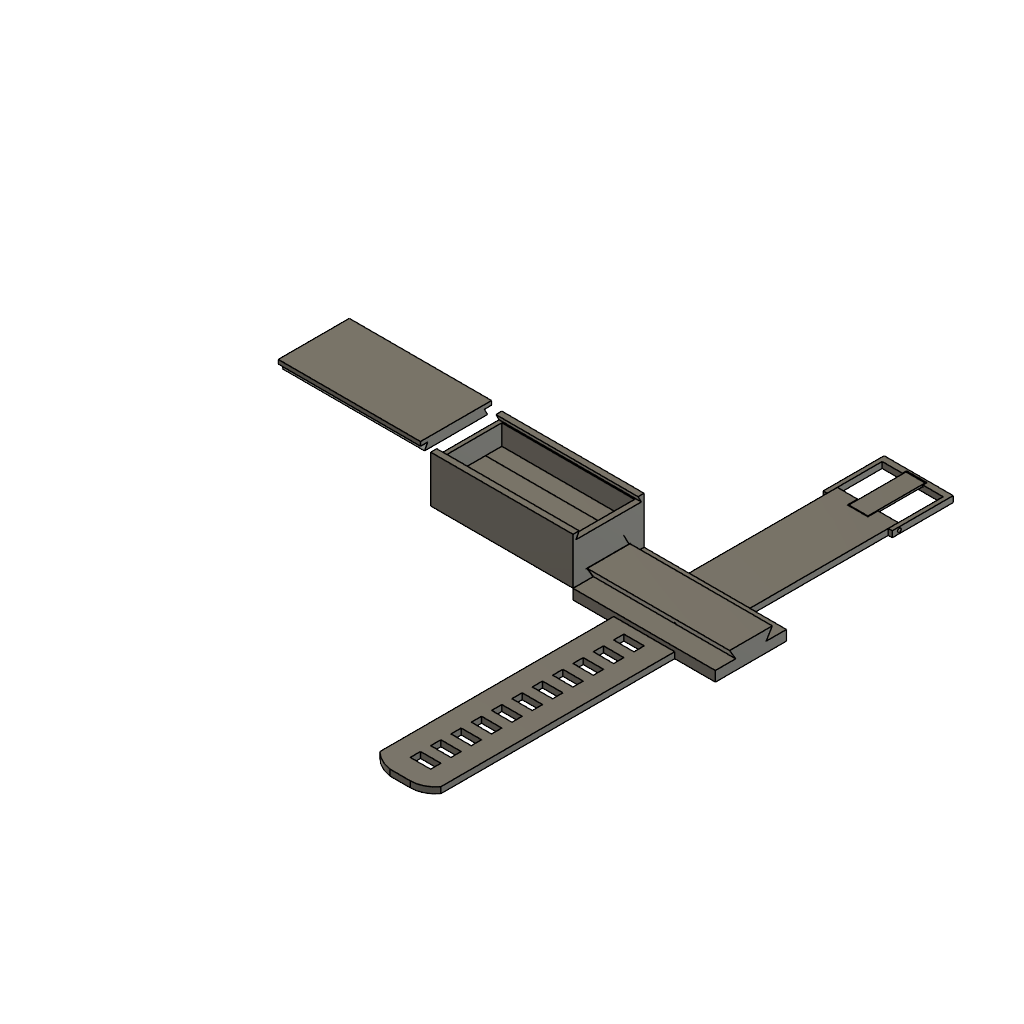
Wristband and components model 2 (Autodesk Fusion 360 design; units mm, degrees)
part number: 2026-09-06-09-34-06-070
Autodesk Fusion 360 part; units mm, degrees
note: some values were not read from the file. Chosen so that the rebuilt part matches the saved one: which bodies a step acts on. Set by a fixed rule: which sketch regions a step uses.
sketch "Sketch1" plane through (0, 0, 0) normal (0, 1, 0) x (1, 0, 0)
  line L0 (0, 35) -> (0, 0)
  line L1 (0, 35) -> (70, 35)
  line L2 (70, 35) -> (70, 0)
  line L3 (70, 0) -> (0, 0)
  constraint vertical L0
  constraint coincident L0.end L3.end
  constraint perpendicular L0 L1
  constraint perpendicular L1 L2
  constraint perpendicular L0 L3
extrude "Extrude1" add sketch "Sketch1" along normal blind 5 makes body 1
sketch "Sketch2" plane through (0, 0, 0) normal (1, 0, 0) x (0, 0, -1)
  line L0 (10, 5) -> (7, 10)
  line L1 (7, 10) -> (28, 10)
  line L2 (28, 10) -> (25, 5)
  line L3 (25, 5) -> (10, 5)
  constraint horizontal L1
  constraint parallel L1 L3
extrude "Extrude2" add sketch "Sketch2" along normal blind 70 bodies 1
sketch "Sketch3" plane through (0, 0, 0) normal (1, 0, 0) x (0, 0, -1)
  line L0 (9.85, 5) -> (6.9, 10)
  line L1 (6.9, 10) -> (6.4, 10.1)
  line L2 (6.4, 10.1) -> (28.25, 10.1)
  line L3 (28.25, 10.1) -> (28.05, 10)
  line L4 (28.05, 10) -> (25.177, 5.0231)
  line L5 (25.177, 5.0231) -> (35, 5.0231)
  line L6 (35, 5.0231) -> (35, 15)
  line L7 (35, 15) -> (0, 15)
  line L8 (0, 15) -> (0, 5.0231)
  line L9 (0, 5.0231) -> (9.85, 5)
  constraint horizontal L2
  constraint parallel L2 L5
  constraint perpendicular L2 L6
  constraint perpendicular L6 L7
  constraint perpendicular L7 L8
extrude "Extrude3" add sketch "Sketch3" against normal blind 70 separate body makes body 2
move_body "Move1" bodies 2 to x (1, 0, 0) y (0, 1, 0) z (0, 0, 1) at (-9, 0, 0)
move_body "Move2" bodies 2 to x (1, 0, 0) y (0, 1, 0) z (0, 0, 1) at (79, 0, 0)
ref_plane "WorkPlane1" through (0, 5, 0) normal (0, 1, 0) x (0, 0, 1)
sketch "Sketch4" plane through (0, 5, 0) normal (0, 1, 0) x (1, 0, 0)
  arc A0 (40, 10) -> (40.5, 9.5) centre (40.6858, 10.1858) ccw
  arc A1 (40.5, 9.5) -> (40.9, 10) centre (40.2285, 10.1272) ccw
  line L0 (40, 10) -> (40.9, 10)
  constraint horizontal L0
extrude "Extrude4" cut sketch "Sketch4" along normal blind 1 bodies 1 2
move_body "Move3" bodies 2 to x (1, 0, 0) y (0, 1, 0) z (0, 0, 1) at (-75, 0, 0)
sketch "Sketch5" plane through (0, 0, 0) normal (1, 0, 0) x (0, 0, -1)
  line L0 (7.5, 10.1) -> (10, 15)
  line L1 (10, 15) -> (25, 15)
  line L2 (25, 15) -> (27.5, 10.1)
  line L3 (27.5, 10.1) -> (7.5, 10.1)
  constraint horizontal L1
  constraint parallel L1 L3
extrude "Extrude5" cut sketch "Sketch5" against normal blind 75 bodies 2 makes body 3 at (-28.3333, 15, -6.6667)
sketch "Sketch7" plane through (0, 0, 0) normal (1, 0, 0) x (0, 0, -1)
  line L0 (0, 25) -> (35, 25)
  line L1 (27.5, 10.1) -> (7.5, 10.1)
  line L2 (7.5, 10.1) -> (10, 15)
  line L3 (10, 15) -> (0, 15)
  line L4 (0, 15) -> (0, 25)
  line L5 (35, 25) -> (35, 14.9709)
  line L6 (35, 14.9709) -> (25, 14.9709)
  line L7 (25, 14.9709) -> (27.5, 10.1)
  constraint perpendicular L0 L4
  constraint perpendicular L0 L5
  constraint perpendicular L5 L6
move_body "Move4" bodies 2 3 to x (1, 0, 0) y (0, 1, 0) z (0, 0, 1) at (5, 0, 0)
extrude "Extrude6" add sketch "Sketch7" against normal blind 70 bodies 1 3
combine "Combine1" operation add target body 3 tool bodies 2
sketch "Sketch8" plane through (0, 25, 0) normal (0, 1, 0) x (-1, 0, 0)
  line L0 (0, 0) -> (0, -35)
  line L1 (0, -35) -> (70, -35)
  line L2 (70, -35) -> (70, 0)
  line L3 (70, 0) -> (0, 0)
  line L4 (68, -33) -> (2.749, -33)
  line L5 (2.749, -33) -> (2.749, -2.8)
  line L6 (2.749, -2.8) -> (68, -2.8)
  line L7 (68, -2.8) -> (68, -33)
  dimension "d16" = 30.2
  constraint horizontal L4
  constraint vertical L5
  constraint horizontal L6
  constraint vertical L7
  measures "d16" distance of L4.start L6.end
extrude "Extrude7" cut sketch "Sketch8" against normal blind 10 contours L4 L5 L6 L7 bodies 3
sketch "Sketch9" plane through (0, 0, 0) normal (1, 0, 0) x (0, 0, -1)
  line L0 (0, 25) -> (0, 28)
  line L1 (0, 28) -> (3, 28)
  line L2 (3, 28) -> (1.5, 25)
  line L3 (1.5, 25) -> (0, 25)
  line L4 (35, 25) -> (35, 28)
  line L5 (35, 28) -> (32, 28)
  line L6 (32, 28) -> (33.6009, 25)
  line L7 (33.6009, 25) -> (35, 25)
  constraint vertical L0
  constraint perpendicular L0 L1
  constraint perpendicular L0 L3
  constraint perpendicular L3 L4
  constraint perpendicular L4 L5
  constraint perpendicular L4 L7
extrude "Extrude8" add sketch "Sketch9" against normal blind 70 bodies 3
sketch "Sketch12" plane through (0, 0, 0) normal (1, 0, 0) x (0, 0, -1)
  line L0 (2, 25) -> (3.5, 28)
  line L1 (3.5, 28) -> (0, 28)
  line L2 (0, 28) -> (0, 30)
  line L3 (0, 30) -> (35, 30)
  line L4 (35, 30) -> (35, 28)
  line L5 (35, 28) -> (31.5, 28)
  line L6 (31.5, 28) -> (33, 25)
  line L7 (33, 25) -> (2, 25)
  constraint horizontal L1
  constraint perpendicular L1 L2
  constraint perpendicular L2 L3
  constraint perpendicular L3 L4
  constraint perpendicular L4 L5
  constraint perpendicular L4 L7
extrude "Extrude9" add sketch "Sketch12" against normal blind 70 separate body makes body 4
move_body "Move5" bodies 4 to x (1, 0, 0) y (0, 1, 0) z (0, 0, 1) at (70, 0, 0)
move_body "Move6" bodies 4 to x (1, 0, 0) y (0, 1, 0) z (0, 0, 1) at (-145, 0, 0)
sketch "Sketch13" plane through (0, 0, 0) normal (0, 1, 0) x (1, 0, 0)
  line L0 (20, 0) -> (50, 0)
  line L1 (50, 0) -> (50, -120)
  line L2 (50, -120) -> (20, -120)
  line L3 (20, -120) -> (20, 0)
  line L4 (20, 35) -> (50, 35)
  line L5 (50, 35) -> (50, 110)
  line L6 (50, 110) -> (20, 110)
  line L7 (20, 110) -> (20, 35)
  constraint horizontal L0
  constraint vertical L1
  constraint horizontal L2
  constraint vertical L3
  constraint horizontal L4
  constraint vertical L5
  constraint horizontal L6
  constraint vertical L7
extrude "Extrude10" add sketch "Sketch13" along normal blind 3 bodies 1
sketch "Sketch14" plane through (0, 3, 0) normal (0, 1, 0) x (-1, 0, 0)
  line L0 (-40.9, -10) -> (-40, -10)
  line L1 (-40, -10) -> (0, -10)
  line L2 (0, -10) -> (0, 0)
  line L3 (0, 0) -> (-70, 0)
  line L4 (-70, 0) -> (-70, -10)
  line L5 (-30, 5) -> (-40, 5)
  line L6 (-40, 5) -> (-40, 10)
  line L7 (-40, 10) -> (-30, 10)
  line L8 (-30, 10) -> (-30, 5)
  line L9 (-30, 15) -> (-40, 15)
  line L10 (-40, 15) -> (-40, 20)
  line L11 (-40, 20) -> (-30, 20)
  line L12 (-30, 20) -> (-30, 15)
  line L13 (-30, 25) -> (-40, 25)
  line L14 (-40, 25) -> (-40, 30)
  line L15 (-40, 30) -> (-30, 30)
  line L16 (-30, 30) -> (-30, 25)
  line L17 (-30, 35) -> (-40, 35)
  line L18 (-40, 35) -> (-40, 40)
  line L19 (-40, 40) -> (-30, 40)
  line L20 (-30, 40) -> (-30, 35)
  line L21 (-30, 45) -> (-40, 45)
  line L22 (-40, 45) -> (-40, 50)
  line L23 (-40, 50) -> (-30, 50)
  line L24 (-30, 50) -> (-30, 45)
  line L25 (-30, 55) -> (-40, 55)
  line L26 (-40, 55) -> (-40, 60)
  line L27 (-40, 60) -> (-30, 60)
  line L28 (-30, 60) -> (-30, 55)
  line L29 (-30, 65) -> (-40, 65)
  line L30 (-40, 65) -> (-40, 70)
  line L31 (-40, 70) -> (-30, 70)
  line L32 (-30, 70) -> (-30, 65)
  line L33 (-30, 75) -> (-40, 75)
  line L34 (-40, 75) -> (-40, 80)
  line L35 (-40, 80) -> (-30, 80)
  line L36 (-30, 80) -> (-30, 75)
  line L37 (-30, 85) -> (-40, 85)
  line L38 (-40, 85) -> (-40, 90)
  line L39 (-40, 90) -> (-30, 90)
  line L40 (-30, 90) -> (-30, 85)
  line L41 (-30, 95) -> (-40, 95)
  line L42 (-40, 95) -> (-40, 100)
  line L43 (-40, 100) -> (-30, 100)
  line L44 (-30, 100) -> (-30, 95)
  line L45 (-30, 105) -> (-40, 105)
  line L46 (-40, 105) -> (-40, 110)
  line L47 (-40, 110) -> (-30, 110)
  line L48 (-30, 110) -> (-30, 105)
  arc A0 (-20, 115) -> (-30, 120) centre (-32.5, 102.5) ccw
  line L49 (-20, 115) -> (-20, 120)
  line L50 (-40, 120) -> (-50, 120)
  arc A1 (-39, 120) -> (-50, 115) centre (-37.9615, 103.1154) ccw
  line L51 (-70, -10) -> (-40.9, -10)
  constraint perpendicular L5 L6
  constraint perpendicular L5 L8
  constraint horizontal L9
  constraint vertical L10
  constraint horizontal L11
  constraint vertical L12
  constraint horizontal L13
  constraint vertical L14
  constraint horizontal L15
  constraint vertical L16
  constraint horizontal L17
  constraint vertical L18
  constraint horizontal L19
  constraint vertical L20
  constraint horizontal L21
  constraint vertical L22
  constraint horizontal L23
  constraint vertical L24
  constraint horizontal L25
  constraint vertical L26
  constraint horizontal L27
  constraint vertical L28
  constraint horizontal L29
  constraint vertical L30
  constraint horizontal L31
  constraint vertical L32
  constraint horizontal L33
  constraint vertical L34
  constraint horizontal L35
  constraint vertical L36
  constraint horizontal L37
  constraint vertical L38
  constraint horizontal L39
  constraint vertical L40
  constraint horizontal L41
  constraint vertical L42
  constraint horizontal L43
  constraint vertical L44
  constraint horizontal L45
  constraint vertical L46
  constraint horizontal L47
  constraint vertical L48
extrude "Extrude11" cut sketch "Sketch14" against normal blind 17 contours L5 L6 L7 L8 | L9 L10 L11 L12 | L13 L14 L15 L16 | L17 L18 L19 L20 | L21 L22 L23 L24 | L25 L26 L27 L28 | L29 L30 L31 L32 | L33 L34 L35 L36 | L37 L38 L39 L40 | L41 L42 L43 L44 | L45 L46 L47 L48 bodies 1
sketch "Sketch15" plane through (0, 0, 0) normal (0, 1, 0) x (1, 0, 0)
  line L0 (20, -120) -> (30, -120)
  arc A0 (20, -115) -> (30, -120) centre (32.5, -102.5) ccw
  line L1 (20, -115) -> (20, -120)
  line L2 (50, -115) -> (50, -120)
  line L3 (50, -120) -> (40, -120)
  arc A1 (40, -120) -> (50, -115) centre (40, -107.5) ccw
  constraint horizontal L0
  constraint perpendicular L0 L1
  constraint perpendicular L0 L2
  constraint perpendicular L2 L3
  constraint tangent L3 A1
extrude "Extrude12" cut sketch "Sketch15" along normal blind 130 bodies 1
sketch "Sketch16" plane through (0, 0, 0) normal (0, 1, 0) x (1, 0, 0)
  line L0 (50, 105) -> (52, 105)
  line L1 (52, 105) -> (52, 135)
  line L2 (52, 135) -> (18, 135)
  line L3 (18, 135) -> (18, 105)
  line L4 (18, 105) -> (20, 105)
  line L5 (20, 105) -> (20, 111)
  line L6 (20, 111) -> (50, 111)
  line L7 (50, 111) -> (50, 105)
  constraint horizontal L0
  constraint perpendicular L0 L1
  constraint perpendicular L1 L2
  constraint perpendicular L2 L3
  constraint perpendicular L3 L4
  constraint perpendicular L4 L5
  constraint perpendicular L5 L6
  constraint perpendicular L0 L7
extrude "Extrude13" add sketch "Sketch16" along normal blind 3 separate body makes body 5
sketch "Sketch18" plane through (0, 0, 0) normal (0, 1, 0) x (1, 0, 0)
  line L0 (50, 111) -> (20, 111)
  line L1 (20, 111) -> (20, 132)
  line L2 (20, 132) -> (50, 132)
  line L3 (50, 132) -> (50, 111)
  constraint horizontal L0
  constraint vertical L1
  constraint horizontal L2
  constraint vertical L3
extrude "Extrude14" cut sketch "Sketch18" along normal blind 100 bodies 5
sketch "Sketch19" plane through (0, 0, 0) normal (0, 1, 0) x (1, 0, 0)
  line L0 (38, 132, 3) -> (30, 132, 3)
  line L1 (30, 132, 3) -> (30, 134, 3)
  line L2 (30, 134, 3) -> (38, 134, 3)
  line L3 (38, 134, 3) -> (38, 132, 3)
sketch "Sketch19 (curves 3 mm off its plane)" plane through (0, 3, 0) normal (0, 1, 0) x (1, 0, 0)
  line L0 (38, 132) -> (30, 132)
  line L1 (30, 132) -> (30, 134)
  line L2 (30, 134) -> (38, 134)
  line L3 (38, 134) -> (38, 132)
extrude "Extrude15" cut sketch "Sketch19 (curves 3 mm off its plane)" against normal blind 1 bodies 5
sketch "Sketch20" plane through (0, 0, 0) normal (0, 1, 0) x (1, 0, 0)
  line L0 (38, 133, 3) -> (30, 133, 3)
  line L1 (30, 133, 3) -> (30, 105, 3)
  line L2 (30, 105, 3) -> (38, 105, 3)
  line L3 (38, 105, 3) -> (38, 133, 3)
sketch "Sketch20 (curves 3 mm off its plane)" plane through (0, 3, 0) normal (0, 1, 0) x (1, 0, 0)
  line L0 (38, 133) -> (30, 133)
  line L1 (30, 133) -> (30, 105)
  line L2 (30, 105) -> (38, 105)
  line L3 (38, 105) -> (38, 133)
extrude "Extrude16" cut sketch "Sketch20 (curves 3 mm off its plane)" against normal blind 1 bodies 1
extrude "Extrude17" cut 1 faces at (35.3333, 2, -106.6667) along direction (0, -1, 0) blind 13 on bodies 1 bodies 1
extrude "Extrude18" cut 1 faces at (38, 2, -106.6667) along direction (1, 0, 0) blind 2 on bodies 1 bodies 1
extrude "Extrude19" cut 1 faces at (38, 2.6667, -133.3333) along direction (1, 0, 0) blind 2 on bodies 5 bodies 5
sketch "Sketch21" plane through (0, 0, 0) normal (0, 1, 0) x (1, 0, 0)
  line L0 (39.7, 105.3) -> (30.3, 105.3)
  line L1 (30.3, 105.3) -> (30.3, 110)
  line L2 (30.3, 110) -> (39.7, 110)
  line L3 (39.7, 110) -> (39.7, 105.3)
  constraint horizontal L0
  constraint vertical L1
  constraint horizontal L2
  constraint vertical L3
extrude "Extrude20" add sketch "Sketch21" along normal blind 2 separate body makes body 6
sketch "Sketch22" plane through (0, 2, 0) normal (0, 1, 0) x (-1, 0, 0)
  line L0 (-39.7, -110) -> (-30.3, -110)
  line L1 (-30.3, -110) -> (-30.3, -105.3)
  line L2 (-30.3, -105.3) -> (-39.7, -105.3)
  line L3 (-39.7, -105.3) -> (-39.7, -110)
  line L4 (-39.7, -105.3) -> (-30.3, -105.3)
  line L5 (-30.3, -105.3) -> (-30.3, -133.4326)
  line L6 (-30.3, -133.4326) -> (-39.7, -133.4326)
  line L7 (-39.7, -133.4326) -> (-39.7, -105.3)
  constraint horizontal L4
  constraint vertical L5
  constraint horizontal L6
  constraint vertical L7
  constraint coincident L2.end L3.start
extrude "Extrude21" add sketch "Sketch22" along normal blind 1 bodies 5 6
sketch "Sketch23" plane through (0, 0, 0) normal (1, 0, 0) x (0, 0, -1)
  circle A0 centre (108.5, 1.5) radius 0.9
  dimension "d47" = 1.8
  measures "d47" diameter of A0
extrude "Extrude22" cut sketch "Sketch23" along normal blind 65 bodies 1 5
named bodies: "TPU wristband", "Components box", "Lid"
